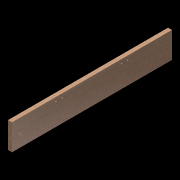
# Autodesk Inventor part: Bumper Wood Side
Saved by Autodesk Inventor 2014 SP1 (Build 180222100, 222)
## iProperties
Created: 2013-11-29
Part Number: Bumper Wood Side
Material: Oak, White
Document SubType Name: Modeling
Designer: Rauhul Varma
Mass: 1360.69 g
Surface Area: 2342.5 cm^2
Volume: 1887.22 cm^3
Density: 0.721 g/cm^3
Appearance: White Oak - Solid Natural Medium Gloss
Author: Rauhul Varma
Autodesk Inventor part; units mm, degrees
ref_plane "YZ Plane" through (0, 0, 0) normal (1, 0, 0) x (0, 1, 0)
ref_plane "XZ Plane" through (0, 0, 0) normal (0, 1, 0) x (-1, 0, 0)
ref_plane "XY Plane" through (0, 0, 0) normal (0, 0, 1) x (1, 0, 0)
sketch "Sketch1" plane through (0, 0, 0) normal (0, 0, 1) x (1, 0, 0)
  line L0 (0, 0) -> (19.05, 0)
  line L1 (19.05, 0) -> (19.05, 127)
  line L2 (19.05, 127) -> (0, 127)
  line L3 (0, 127) -> (0, 0)
  dimension "d0" = 19.05
  dimension "d1" = 127
  constraints: 8 end point, 2 parallel, 1 horizontal, 1 perpendicular
  measures "d0" distance of L2.end L1.end
  measures "d1" distance of L1.end L0.end
extrude "Extrusion1" add sketch "Sketch1" along normal blind 781.05
sketch "Sketch2" plane through (19.05, 0, 0) normal (1, 0, 0) x (0, 0, -1)
  line L0 (0, 0) -> (0, 127) projected
  line L1 (0, 127) -> (-781.05, 127) projected
  line L2 (-781.05, 0) -> (-781.05, 127) projected
  line L3 (0, 0) -> (-781.05, 0) projected
  line L4 (-781.05, 107.95) -> (0, 107.95) construction
  point P0 (-565.6552, 107.95)
  point P1 (-535.6552, 107.95)
  point P2 (-215.3948, 107.95)
  point P3 (-245.3948, 107.95)
  dimension "d4" = 19.05
  dimension "d5" = 215.3948
  dimension "d6" = 30
  dimension "d7" = 30
  dimension "d8" = 215.3948
  constraints: 6 point on line, 2 end point, 1 parallel
  measures "d4" distance between parallel lines of L1 L4
  measures "d5" distance from line of L2 point (-565.655, 107.95)
  measures "d6" distance of point (-535.655, 107.95) point (-565.655, 107.95)
  measures "d7" distance of point (-215.395, 107.95) point (-245.395, 107.95)
  measures "d8" distance from line of L0 point (-215.395, 107.95)
hole "Hole1" at (19.05, 107.95, 565.6552) at (19.05, 107.95, 535.6552) at (19.05, 107.95, 215.3948) at (19.05, 107.95, 245.3948) direction (-1, 0, 0) diameter 6.35 end through all
equation "\"d7\" = d6"
equation "\"d8\" = d5"
body "Solid1"
